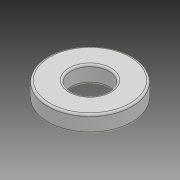
# Autodesk Inventor part: bearing
Saved by Autodesk Inventor 2018 (Build 220112000, 112)
## iProperties
Created: 2019-02-20
Part Number: bearing
Material: 一般
Document SubType Name: Modeling
Designer: ku_sk
Density: 1 g/cm^3
Appearance: 既定
Author: ku_sk
Autodesk Inventor part; units mm, degrees
ref_plane "YZ Plane" through (0, 0, 0) normal (1, 0, 0) x (0, 1, 0)
ref_plane "XZ Plane" through (0, 0, 0) normal (0, 1, 0) x (-1, 0, 0)
ref_plane "XY Plane" through (0, 0, 0) normal (0, 0, 1) x (1, 0, 0)
sketch "スケッチ1" plane through (0, 0, 0) normal (0, 0, 1) x (1, 0, 0)
  circle A0 centre (0, 0) radius 7.9375
  circle A1 centre (0, 0) radius 17.4625
  dimension "d0" = 15.875
  dimension "d1" = 34.925
  constraints: 2 centre point, 2 coincident
  measures "d0" diameter of A0
  measures "d1" diameter of A1
extrude "押し出し1" add sketch "スケッチ1" along normal mid plane 7.142
fillet "フィレット1" radius 0.8 4 edges at (-17.4625, 0, 3.571) (-17.4625, 0, -3.571) (-7.9375, 0, 3.571) (-7.9375, 0, -3.571)
